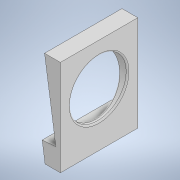
# Autodesk Inventor part: exhastForGasVent02
Saved by Autodesk Inventor 2021.1 (Build 251245000, 245)
## iProperties
Created: 2020-08-27
Part Number: exhastForGasVent02
Material: Generic
Document SubType Name: Modeling
Designer: robst
Density: 1 g/cm^3
Appearance: Default
Author: robst
Autodesk Inventor part; units mm, degrees
ref_plane "YZ Plane" through (0, 0, 0) normal (1, 0, 0) x (0, 1, 0)
ref_plane "XZ Plane" through (0, 0, 0) normal (0, 1, 0) x (-1, 0, 0)
ref_plane "XY Plane" through (0, 0, 0) normal (0, 0, 1) x (1, 0, 0)
sketch "Sketch6" plane through (0, 0, 0) normal (0, 0, 1) x (1, 0, 0)
  line L0 (0, 0) -> (0, 83.82)
  line L1 (0, 83.82) -> (-17.653, 83.82)
  line L2 (-17.653, 83.82) -> (-5.08, 0)
  line L3 (0, 0) -> (0, -22.86)
  line L4 (0, -22.86) -> (-17.091, -22.86)
  line L5 (-23.2881, 0) -> (-5.08, 0) construction
  line L6 (-5.08, 0) -> (-20.32, -1.3333)
  line L7 (-20.32, -1.3333) -> (-17.091, -22.86)
  dimension "d31" = 83.82
  dimension "d32" = 17.653
  dimension "d33" = 22.86
  dimension "d35" = 5
  dimension "d36" = 0
  dimension "d37" = 5.08
  dimension "d47" = 20.32
  constraints: 16 end point, 2 parallel, 2 perpendicular, 2 vertical
  measures "d31" distance of L0.start L0.end
  measures "d32" distance of L0.end L1.end
  measures "d33" distance of L0.start L3.end
  measures "d35" angle of L6 L5
  measures "d36" vertical distance of L2.end L0.start
  measures "d37" distance of L2.end L0.start
  measures "d47" distance from line of L6.end L3
extrude "Extrusion7" add sketch "Sketch6" along normal mid plane 86.36
sketch "Sketch7" plane through (0, -22.86, 43.18) normal (1, 0, 0) x (0, 0, -1)
  line L0 (86.36, 22.86) -> (0, 22.86) projected
  line L1 (0, 106.68) -> (86.36, 106.68) construction
  line L2 (43.18, 106.68) -> (43.18, 22.86) construction
  circle A0 centre (43.18, 59.69) radius 31.75
  dimension "d40" = 63.5
  dimension "d41" = 5.08
  constraints: 2 end point, 1 centre point, 1 midpoint, 1 perpendicular, 1 point on line
  measures "d40" diameter of A0
  measures "d41" distance edge to line of A0 L0
extrude "Extrusion8" cut sketch "Sketch7" against normal through all
sketch "Sketch11" plane through (-17.091, -22.86, -43.18) normal (-0.9889364, -0.1483405, 0) x (0, 0, 1)
  line L0 (43.18, 20.0718) -> (43.18, 0) construction
  line L1 (0, 0) -> (86.36, 0) construction
  line L2 (43.18, 10.0359) -> (86.36, 10.0359) construction
  spline S0 degree 2 poles (51.8782, 10.9729) (51.4467, 10.9729) (50.7321, 11.2363) (50.4752, 11.5031) knots 0 0 0 1 2 2 2
  spline S1 degree 2 poles (50.4752, 11.5031) (50.2183, 11.7731) (49.945, 12.5701) (49.945, 13.0872) knots 0 0 0 1 2 2 2
  spline S2 degree 2 poles (49.945, 13.0872) (49.945, 13.5779) (50.2216, 14.3551) (50.4785, 14.6318) knots 0 0 0 1 2 2 2
  spline S3 degree 2 poles (50.4785, 14.6318) (50.7255, 14.8985) (51.45, 15.1884) (51.8815, 15.1884) knots 0 0 0 1 2 2 2
  spline S4 degree 2 poles (51.8815, 15.1884) (52.0889, 15.1884) (52.4644, 15.1291) (52.6356, 15.0764) knots 0 0 0 1 2 2 2
  spline S5 degree 2 poles (52.6356, 15.0764) (52.774, 15.0369) (53.1099, 14.892) (53.212, 14.8393) knots 0 0 0 1 2 2 2
  line L3 (53.212, 14.8393) -> (53.212, 14.1872)
  line L4 (53.212, 14.1872) -> (53.1659, 14.1872)
  spline S6 degree 2 poles (53.1659, 14.1872) (53.0638, 14.2761) (52.8497, 14.4375) (52.6521, 14.5297) knots 0 0 0 1 2 2 2
  spline S7 degree 2 poles (52.6521, 14.5297) (52.4874, 14.612) (52.0626, 14.7207) (51.8189, 14.7207) knots 0 0 0 1 2 2 2
  spline S8 degree 2 poles (51.8189, 14.7207) (51.2327, 14.7207) (50.5081, 13.8381) (50.5081, 13.1037) knots 0 0 0 1 2 2 2
  spline S9 degree 2 poles (50.5081, 13.1037) (50.5081, 12.6953) (50.6991, 12.0827) (50.8803, 11.8719) knots 0 0 0 1 2 2 2
  spline S10 degree 2 poles (50.8803, 11.8719) (51.0548, 11.6612) (51.5488, 11.4405) (51.8584, 11.4405) knots 0 0 0 1 2 2 2
  spline S11 degree 2 poles (51.8584, 11.4405) (52.0856, 11.4405) (52.5401, 11.5064) (52.6949, 11.5722) knots 0 0 0 1 2 2 2
  line L5 (52.6949, 11.5722) -> (52.6949, 12.6228)
  line L6 (52.6949, 12.6228) -> (51.753, 12.6228)
  line L7 (51.753, 12.6228) -> (51.753, 13.0971)
  line L8 (51.753, 13.0971) -> (53.2284, 13.0971)
  line L9 (53.2284, 13.0971) -> (53.2284, 11.322)
  spline S12 degree 2 poles (53.2284, 11.322) (53.1263, 11.2758) (52.7772, 11.1342) (52.629, 11.0914) knots 0 0 0 1 2 2 2
  spline S13 degree 2 poles (52.629, 11.0914) (52.4282, 11.0321) (52.1054, 10.9729) (51.8782, 10.9729) knots 0 0 0 1 2 2 2
  spline S14 degree 2 poles (55.5667, 11.3746) (55.5041, 11.3285) (55.2934, 11.1639) (55.1946, 11.1145) knots 0 0 0 1 2 2 2
  spline S15 degree 2 poles (55.1946, 11.1145) (55.0595, 11.042) (54.806, 10.9663) (54.5754, 10.9663) knots 0 0 0 1 2 2 2
  spline S16 degree 2 poles (54.5754, 10.9663) (54.3877, 10.9663) (54.0485, 11.1079) (53.92, 11.2363) knots 0 0 0 1 2 2 2
  spline S17 degree 2 poles (53.92, 11.2363) (53.7982, 11.3615) (53.65, 11.7303) (53.65, 11.9345) knots 0 0 0 1 2 2 2
  spline S18 degree 2 poles (53.65, 11.9345) (53.65, 12.2507) (53.9167, 12.6986) (54.2066, 12.827) knots 0 0 0 1 2 2 2
  spline S19 degree 2 poles (54.2066, 12.827) (54.4634, 12.9456) (55.1616, 13.0345) (55.5667, 13.0576) knots 0 0 0 1 2 2 2
  line L10 (55.5667, 13.0576) -> (55.5667, 13.1564)
  spline S20 degree 2 poles (55.5667, 13.1564) (55.5667, 13.3342) (55.458, 13.5548) (55.3592, 13.6174) knots 0 0 0 1 2 2 2
  spline S21 degree 2 poles (55.3592, 13.6174) (55.2604, 13.68) (54.9772, 13.7195) (54.8257, 13.7195) knots 0 0 0 1 2 2 2
  spline S22 degree 2 poles (54.8257, 13.7195) (54.6479, 13.7195) (54.167, 13.6141) (53.9266, 13.512) knots 0 0 0 1 2 2 2
  line L11 (53.9266, 13.512) -> (53.897, 13.512)
  line L12 (53.897, 13.512) -> (53.897, 14.0357)
  spline S23 degree 2 poles (53.897, 14.0357) (54.0386, 14.0752) (54.5688, 14.174) (54.829, 14.174) knots 0 0 0 1 2 2 2
  spline S24 degree 2 poles (54.829, 14.174) (55.1452, 14.174) (55.5766, 14.0752) (55.7479, 13.9468) knots 0 0 0 1 2 2 2
  spline S25 degree 2 poles (55.7479, 13.9468) (55.9158, 13.8216) (56.0805, 13.4231) (56.0805, 13.1366) knots 0 0 0 1 2 2 2
  line L13 (56.0805, 13.1366) -> (56.0805, 11.0519)
  line L14 (56.0805, 11.0519) -> (55.5667, 11.0519)
  line L15 (55.5667, 11.0519) -> (55.5667, 11.3746)
  line L16 (55.5667, 11.8028) -> (55.5667, 12.6492)
  spline S26 degree 2 poles (55.5667, 12.6492) (55.3823, 12.6327) (54.8257, 12.5767) (54.6512, 12.524) knots 0 0 0 1 2 2 2
  spline S27 degree 2 poles (54.6512, 12.524) (54.447, 12.4615) (54.1802, 12.2013) (54.1802, 11.9707) knots 0 0 0 1 2 2 2
  spline S28 degree 2 poles (54.1802, 11.9707) (54.1802, 11.7073) (54.4766, 11.4405) (54.7598, 11.4405) knots 0 0 0 1 2 2 2
  spline S29 degree 2 poles (54.7598, 11.4405) (55.0003, 11.4405) (55.3955, 11.648) (55.5667, 11.8028) knots 0 0 0 1 2 2 2
  spline S30 degree 2 poles (57.6251, 10.9794) (57.3188, 10.9794) (56.7886, 11.1441) (56.614, 11.2363) knots 0 0 0 1 2 2 2
  line L17 (56.614, 11.2363) -> (56.614, 11.8127)
  line L18 (56.614, 11.8127) -> (56.6404, 11.8127)
  spline S31 degree 2 poles (56.6404, 11.8127) (56.7062, 11.76) (56.8841, 11.6348) (57.0323, 11.5657) knots 0 0 0 1 2 2 2
  spline S32 degree 2 poles (57.0323, 11.5657) (57.1607, 11.5031) (57.4769, 11.4109) (57.6448, 11.4109) knots 0 0 0 1 2 2 2
  spline S33 degree 2 poles (57.6448, 11.4109) (57.7667, 11.4109) (58.0466, 11.4669) (58.1125, 11.513) knots 0 0 0 1 2 2 2
  spline S34 degree 2 poles (58.1125, 11.513) (58.208, 11.5755) (58.2936, 11.7172) (58.2936, 11.8621) knots 0 0 0 1 2 2 2
  spline S35 degree 2 poles (58.2936, 11.8621) (58.2936, 12.0432) (58.096, 12.2309) (57.8424, 12.2935) knots 0 0 0 1 2 2 2
  spline S36 degree 2 poles (57.8424, 12.2935) (57.7436, 12.3165) (57.4275, 12.3824) (57.2924, 12.4186) knots 0 0 0 1 2 2 2
  spline S37 degree 2 poles (57.2924, 12.4186) (56.9433, 12.5207) (56.6272, 12.9423) (56.6272, 13.242) knots 0 0 0 1 2 2 2
  spline S38 degree 2 poles (56.6272, 13.242) (56.6272, 13.6569) (57.2496, 14.174) (57.7634, 14.174) knots 0 0 0 1 2 2 2
  spline S39 degree 2 poles (57.7634, 14.174) (58.017, 14.174) (58.5307, 14.0489) (58.7053, 13.9533) knots 0 0 0 1 2 2 2
  line L19 (58.7053, 13.9533) -> (58.7053, 13.4034)
  line L20 (58.7053, 13.4034) -> (58.6789, 13.4034)
  spline S40 degree 2 poles (58.6789, 13.4034) (58.4813, 13.5614) (58.0005, 13.7426) (57.7535, 13.7426) knots 0 0 0 1 2 2 2
  spline S41 degree 2 poles (57.7535, 13.7426) (57.4999, 13.7426) (57.1508, 13.5285) (57.1508, 13.3144) knots 0 0 0 1 2 2 2
  spline S42 degree 2 poles (57.1508, 13.3144) (57.1508, 13.1201) (57.3583, 12.9324) (57.5888, 12.8731) knots 0 0 0 1 2 2 2
  spline S43 degree 2 poles (57.5888, 12.8731) (57.7008, 12.8435) (57.984, 12.7842) (58.1388, 12.748) knots 0 0 0 1 2 2 2
  spline S44 degree 2 poles (58.1388, 12.748) (58.4748, 12.6623) (58.8173, 12.2704) (58.8173, 11.9312) knots 0 0 0 1 2 2 2
  spline S45 degree 2 poles (58.8173, 11.9312) (58.8173, 11.7336) (58.6625, 11.3845) (58.511, 11.2561) knots 0 0 0 1 2 2 2
  spline S46 degree 2 poles (58.511, 11.2561) (58.3496, 11.1211) (57.9379, 10.9794) (57.6251, 10.9794) knots 0 0 0 1 2 2 2
  line L21 (64.0273, 15.1159) -> (62.6277, 11.0519)
  line L22 (62.6277, 11.0519) -> (62.0447, 11.0519)
  line L23 (62.0447, 11.0519) -> (60.6451, 15.1159)
  line L24 (60.6451, 15.1159) -> (61.2247, 15.1159)
  line L25 (61.2247, 15.1159) -> (62.351, 11.7402)
  line L26 (62.351, 11.7402) -> (63.4774, 15.1159)
  line L27 (63.4774, 15.1159) -> (64.0273, 15.1159)
  spline S47 degree 2 poles (65.7465, 10.9827) (65.0154, 10.9827) (64.2118, 11.8028) (64.2118, 12.5603) knots 0 0 0 1 2 2 2
  spline S48 degree 2 poles (64.2118, 12.5603) (64.2118, 13.3046) (64.9923, 14.1872) (65.6213, 14.1872) knots 0 0 0 1 2 2 2
  spline S49 degree 2 poles (65.6213, 14.1872) (65.9046, 14.1872) (66.3426, 14.0225) (66.504, 13.848) knots 0 0 0 1 2 2 2
  spline S50 degree 2 poles (66.504, 13.848) (66.6686, 13.6734) (66.8432, 13.1695) (66.8432, 12.804) knots 0 0 0 1 2 2 2
  line L28 (66.8432, 12.804) -> (66.8432, 12.524)
  line L29 (66.8432, 12.524) -> (64.7321, 12.524)
  spline S51 degree 2 poles (64.7321, 12.524) (64.7321, 11.9938) (65.2656, 11.4306) (65.7399, 11.4306) knots 0 0 0 1 2 2 2
  spline S52 degree 2 poles (65.7399, 11.4306) (65.9079, 11.4306) (66.2339, 11.5064) (66.3656, 11.5657) knots 0 0 0 1 2 2 2
  spline S53 degree 2 poles (66.3656, 11.5657) (66.504, 11.6315) (66.695, 11.7468) (66.7575, 11.7995) knots 0 0 0 1 2 2 2
  line L30 (66.7575, 11.7995) -> (66.7872, 11.7995)
  line L31 (66.7872, 11.7995) -> (66.7872, 11.2396)
  spline S54 degree 2 poles (66.7872, 11.2396) (66.6983, 11.2034) (66.4282, 11.098) (66.3228, 11.0684) knots 0 0 0 1 2 2 2
  spline S55 degree 2 poles (66.3228, 11.0684) (66.1746, 11.0256) (65.9309, 10.9827) (65.7465, 10.9827) knots 0 0 0 1 2 2 2
  spline S56 degree 2 poles (66.3426, 12.9159) (66.336, 13.1234) (66.2504, 13.4264) (66.168, 13.5285) knots 0 0 0 1 2 2 2
  spline S57 degree 2 poles (66.168, 13.5285) (66.0791, 13.6438) (65.7992, 13.7656) (65.5917, 13.7656) knots 0 0 0 1 2 2 2
  spline S58 degree 2 poles (65.5917, 13.7656) (65.3875, 13.7656) (65.101, 13.6438) (64.9824, 13.5252) knots 0 0 0 1 2 2 2
  spline S59 degree 2 poles (64.9824, 13.5252) (64.8672, 13.4034) (64.7486, 13.1102) (64.7321, 12.9159) knots 0 0 0 1 2 2 2
  line L32 (64.7321, 12.9159) -> (66.3426, 12.9159)
  line L33 (69.7578, 11.0519) -> (69.244, 11.0519)
  line L34 (69.244, 11.0519) -> (69.244, 12.7908)
  spline S60 degree 2 poles (69.244, 12.7908) (69.244, 13.0016) (69.2045, 13.3638) (69.1452, 13.4725) knots 0 0 0 1 2 2 2
  spline S61 degree 2 poles (69.1452, 13.4725) (69.0826, 13.5878) (68.8587, 13.6998) (68.6677, 13.6998) knots 0 0 0 1 2 2 2
  spline S62 degree 2 poles (68.6677, 13.6998) (68.4767, 13.6998) (68.0716, 13.4956) (67.8773, 13.3309) knots 0 0 0 1 2 2 2
  line L35 (67.8773, 13.3309) -> (67.8773, 11.0519)
  line L36 (67.8773, 11.0519) -> (67.3635, 11.0519)
  line L37 (67.3635, 11.0519) -> (67.3635, 14.1015)
  line L38 (67.3635, 14.1015) -> (67.8773, 14.1015)
  line L39 (67.8773, 14.1015) -> (67.8773, 13.7623)
  spline S63 degree 2 poles (67.8773, 13.7623) (68.1078, 13.9698) (68.5524, 14.1872) (68.8027, 14.1872) knots 0 0 0 1 2 2 2
  spline S64 degree 2 poles (68.8027, 14.1872) (69.2506, 14.1872) (69.7578, 13.5944) (69.7578, 13.0312) knots 0 0 0 1 2 2 2
  line L40 (69.7578, 13.0312) -> (69.7578, 11.0519)
  spline S65 degree 2 poles (71.4012, 10.9926) (70.9829, 10.9926) (70.512, 11.4702) (70.512, 11.9872) knots 0 0 0 1 2 2 2
  line L41 (70.512, 11.9872) -> (70.512, 13.6767)
  line L42 (70.512, 13.6767) -> (70.1662, 13.6767)
  line L43 (70.1662, 13.6767) -> (70.1662, 14.1015)
  line L44 (70.1662, 14.1015) -> (70.512, 14.1015)
  line L45 (70.512, 14.1015) -> (70.512, 14.9776)
  line L46 (70.512, 14.9776) -> (71.0257, 14.9776)
  line L47 (71.0257, 14.9776) -> (71.0257, 14.1015)
  line L48 (71.0257, 14.1015) -> (71.9709, 14.1015)
  line L49 (71.9709, 14.1015) -> (71.9709, 13.6767)
  line L50 (71.9709, 13.6767) -> (71.0257, 13.6767)
  line L51 (71.0257, 13.6767) -> (71.0257, 12.2243)
  spline S66 degree 2 poles (71.0257, 12.2243) (71.0257, 11.9938) (71.0422, 11.7402) (71.0982, 11.6315) knots 0 0 0 1 2 2 2
  spline S67 degree 2 poles (71.0982, 11.6315) (71.1443, 11.536) (71.3518, 11.4405) (71.5296, 11.4405) knots 0 0 0 1 2 2 2
  spline S68 degree 2 poles (71.5296, 11.4405) (71.6548, 11.4405) (71.8886, 11.5163) (71.9413, 11.5393) knots 0 0 0 1 2 2 2
  line L52 (71.9413, 11.5393) -> (71.9709, 11.5393)
  line L53 (71.9709, 11.5393) -> (71.9709, 11.0782)
  spline S69 degree 2 poles (71.9709, 11.0782) (71.826, 11.0387) (71.5296, 10.9926) (71.4012, 10.9926) knots 0 0 0 1 2 2 2
  spline S70 degree 2 poles (76.5487, 13.0839) (76.5487, 11.9905) (75.9131, 10.9663) (75.2511, 10.9663) knots 0 0 0 1 2 2 2
  spline S71 degree 2 poles (75.2511, 10.9663) (74.5793, 10.9663) (73.9502, 12.0103) (73.9502, 13.0806) knots 0 0 0 1 2 2 2
  spline S72 degree 2 poles (73.9502, 13.0806) (73.9502, 14.1806) (74.5858, 15.1982) (75.2511, 15.1982) knots 0 0 0 1 2 2 2
  spline S73 degree 2 poles (75.2511, 15.1982) (75.9197, 15.1982) (76.5487, 14.1444) (76.5487, 13.0839) knots 0 0 0 1 2 2 2
  spline S74 degree 2 poles (75.8505, 11.8456) (75.9295, 12.0465) (75.9954, 12.6656) (75.9954, 13.0839) knots 0 0 0 1 2 2 2
  spline S75 degree 2 poles (75.9954, 13.0839) (75.9954, 13.5022) (75.9295, 14.118) (75.8472, 14.3255) knots 0 0 0 1 2 2 2
  spline S76 degree 2 poles (75.8472, 14.3255) (75.7649, 14.533) (75.4783, 14.747) (75.2511, 14.747) knots 0 0 0 1 2 2 2
  spline S77 degree 2 poles (75.2511, 14.747) (75.0239, 14.747) (74.7308, 14.533) (74.6451, 14.3189) knots 0 0 0 1 2 2 2
  spline S78 degree 2 poles (74.6451, 14.3189) (74.5628, 14.1114) (74.5035, 13.4791) (74.5035, 13.0806) knots 0 0 0 1 2 2 2
  spline S79 degree 2 poles (74.5035, 13.0806) (74.5035, 12.6525) (74.5562, 12.0794) (74.6418, 11.8555) knots 0 0 0 1 2 2 2
  spline S80 degree 2 poles (74.6418, 11.8555) (74.7209, 11.6447) (75.014, 11.4175) (75.2511, 11.4175) knots 0 0 0 1 2 2 2
  spline S81 degree 2 poles (75.2511, 11.4175) (75.475, 11.4175) (75.7682, 11.6315) (75.8505, 11.8456) knots 0 0 0 1 2 2 2
  line L54 (79.5753, 11.0519) -> (77.069, 11.0519)
  line L55 (77.069, 11.0519) -> (77.069, 11.6282)
  spline S82 degree 2 poles (77.069, 11.6282) (77.3391, 11.8818) (77.8199, 12.3528) (78.0505, 12.6064) knots 0 0 0 1 2 2 2
  spline S83 degree 2 poles (78.0505, 12.6064) (78.5148, 13.1168) (78.854, 13.7294) (78.854, 14.0554) knots 0 0 0 1 2 2 2
  spline S84 degree 2 poles (78.854, 14.0554) (78.854, 14.2267) (78.7486, 14.4836) (78.6531, 14.5659) knots 0 0 0 1 2 2 2
  spline S85 degree 2 poles (78.6531, 14.5659) (78.5576, 14.6482) (78.3073, 14.7306) (78.1558, 14.7306) knots 0 0 0 1 2 2 2
  spline S86 degree 2 poles (78.1558, 14.7306) (78.0109, 14.7306) (77.7145, 14.6581) (77.5795, 14.6021) knots 0 0 0 1 2 2 2
  spline S87 degree 2 poles (77.5795, 14.6021) (77.4642, 14.556) (77.2502, 14.4243) (77.1843, 14.3782) knots 0 0 0 1 2 2 2
  line L56 (77.1843, 14.3782) -> (77.1547, 14.3782)
  line L57 (77.1547, 14.3782) -> (77.1547, 14.9578)
  spline S88 degree 2 poles (77.1547, 14.9578) (77.3226, 15.0402) (77.9253, 15.2015) (78.1954, 15.2015) knots 0 0 0 1 2 2 2
  spline S89 degree 2 poles (78.1954, 15.2015) (78.7651, 15.2015) (79.4073, 14.5988) (79.4073, 14.0851) knots 0 0 0 1 2 2 2
  spline S90 degree 2 poles (79.4073, 14.0851) (79.4073, 13.8447) (79.2953, 13.4429) (79.1965, 13.2716) knots 0 0 0 1 2 2 2
  spline S91 degree 2 poles (79.1965, 13.2716) (79.0977, 13.0938) (78.8112, 12.7447) (78.6531, 12.5767) knots 0 0 0 1 2 2 2
  spline S92 degree 2 poles (78.6531, 12.5767) (78.3963, 12.2968) (77.7672, 11.6974) (77.5795, 11.5228) knots 0 0 0 1 2 2 2
  line L58 (77.5795, 11.5228) -> (79.5753, 11.5228)
  line L59 (79.5753, 11.5228) -> (79.5753, 11.0519)
  spline S93 degree 2 poles (55.4646, 7.1796) (55.4646, 6.9162) (55.2769, 6.4419) (55.1089, 6.2773) knots 0 0 0 1 2 2 2
  spline S94 degree 2 poles (55.1089, 6.2773) (54.8982, 6.0698) (54.3284, 5.8557) (53.8937, 5.8557) knots 0 0 0 1 2 2 2
  line L60 (53.8937, 5.8557) -> (53.4359, 5.8557)
  line L61 (53.4359, 5.8557) -> (53.4359, 4.3408)
  line L62 (53.4359, 4.3408) -> (52.8958, 4.3408)
  line L63 (52.8958, 4.3408) -> (52.8958, 8.4048)
  line L64 (52.8958, 8.4048) -> (53.9167, 8.4048)
  spline S95 degree 2 poles (53.9167, 8.4048) (54.279, 8.4048) (54.7862, 8.2862) (54.9805, 8.1512) knots 0 0 0 1 2 2 2
  spline S96 degree 2 poles (54.9805, 8.1512) (55.2077, 7.9964) (55.4646, 7.5189) (55.4646, 7.1796) knots 0 0 0 1 2 2 2
  spline S97 degree 2 poles (54.9015, 7.1632) (54.9015, 7.374) (54.7566, 7.6835) (54.6084, 7.7823) knots 0 0 0 1 2 2 2
  spline S98 degree 2 poles (54.6084, 7.7823) (54.4799, 7.868) (54.1374, 7.9371) (53.8838, 7.9371) knots 0 0 0 1 2 2 2
  line L65 (53.8838, 7.9371) -> (53.4359, 7.9371)
  line L66 (53.4359, 7.9371) -> (53.4359, 6.3168)
  line L67 (53.4359, 6.3168) -> (53.8048, 6.3168)
  spline S99 degree 2 poles (53.8048, 6.3168) (54.1341, 6.3168) (54.5392, 6.4222) (54.6709, 6.5605) knots 0 0 0 1 2 2 2
  spline S100 degree 2 poles (54.6709, 6.5605) (54.7928, 6.6824) (54.9015, 6.9689) (54.9015, 7.1632) knots 0 0 0 1 2 2 2
  line L68 (57.5559, 6.8404) -> (57.5296, 6.8404)
  spline S101 degree 2 poles (57.5296, 6.8404) (57.4703, 6.8569) (57.3418, 6.8635) (57.2529, 6.8635) knots 0 0 0 1 2 2 2
  spline S102 degree 2 poles (57.2529, 6.8635) (57.0454, 6.8635) (56.6371, 6.6824) (56.4526, 6.5045) knots 0 0 0 1 2 2 2
  line L69 (56.4526, 6.5045) -> (56.4526, 4.3408)
  line L70 (56.4526, 4.3408) -> (55.9389, 4.3408)
  line L71 (55.9389, 4.3408) -> (55.9389, 7.3904)
  line L72 (55.9389, 7.3904) -> (56.4526, 7.3904)
  line L73 (56.4526, 7.3904) -> (56.4526, 6.9359)
  spline S103 degree 2 poles (56.4526, 6.9359) (56.7326, 7.1862) (57.1508, 7.3904) (57.3484, 7.3904) knots 0 0 0 1 2 2 2
  spline S104 degree 2 poles (57.3484, 7.3904) (57.4275, 7.3904) (57.5065, 7.3838) (57.5559, 7.374) knots 0 0 0 1 2 2 2
  line L74 (57.5559, 7.374) -> (57.5559, 6.8404)
  line L75 (58.478, 4.3408) -> (57.9643, 4.3408)
  line L76 (57.9643, 4.3408) -> (57.9643, 7.3904)
  line L77 (57.9643, 7.3904) -> (58.478, 7.3904)
  line L78 (58.478, 7.3904) -> (58.478, 4.3408)
  line L79 (58.5143, 7.8976) -> (57.9313, 7.8976)
  line L80 (57.9313, 7.8976) -> (57.9313, 8.4311)
  line L81 (57.9313, 8.4311) -> (58.5143, 8.4311)
  line L82 (58.5143, 8.4311) -> (58.5143, 7.8976)
  line L83 (61.6265, 4.3408) -> (61.1127, 4.3408)
  line L84 (61.1127, 4.3408) -> (61.1127, 6.0797)
  spline S105 degree 2 poles (61.1127, 6.0797) (61.1127, 6.2904) (61.0732, 6.6527) (61.0139, 6.7614) knots 0 0 0 1 2 2 2
  spline S106 degree 2 poles (61.0139, 6.7614) (60.9514, 6.8767) (60.7274, 6.9886) (60.5364, 6.9886) knots 0 0 0 1 2 2 2
  spline S107 degree 2 poles (60.5364, 6.9886) (60.3454, 6.9886) (59.9403, 6.7844) (59.746, 6.6198) knots 0 0 0 1 2 2 2
  line L85 (59.746, 6.6198) -> (59.746, 4.3408)
  line L86 (59.746, 4.3408) -> (59.2322, 4.3408)
  line L87 (59.2322, 4.3408) -> (59.2322, 7.3904)
  line L88 (59.2322, 7.3904) -> (59.746, 7.3904)
  line L89 (59.746, 7.3904) -> (59.746, 7.0512)
  spline S108 degree 2 poles (59.746, 7.0512) (59.9765, 7.2587) (60.4211, 7.476) (60.6714, 7.476) knots 0 0 0 1 2 2 2
  spline S109 degree 2 poles (60.6714, 7.476) (61.1193, 7.476) (61.6265, 6.8832) (61.6265, 6.3201) knots 0 0 0 1 2 2 2
  line L90 (61.6265, 6.3201) -> (61.6265, 4.3408)
  spline S110 degree 2 poles (63.2699, 4.2815) (62.8516, 4.2815) (62.3807, 4.759) (62.3807, 5.2761) knots 0 0 0 1 2 2 2
  line L91 (62.3807, 5.2761) -> (62.3807, 6.9656)
  line L92 (62.3807, 6.9656) -> (62.0349, 6.9656)
  line L93 (62.0349, 6.9656) -> (62.0349, 7.3904)
  line L94 (62.0349, 7.3904) -> (62.3807, 7.3904)
  line L95 (62.3807, 7.3904) -> (62.3807, 8.2665)
  line L96 (62.3807, 8.2665) -> (62.8944, 8.2665)
  line L97 (62.8944, 8.2665) -> (62.8944, 7.3904)
  line L98 (62.8944, 7.3904) -> (63.8396, 7.3904)
  line L99 (63.8396, 7.3904) -> (63.8396, 6.9656)
  line L100 (63.8396, 6.9656) -> (62.8944, 6.9656)
  line L101 (62.8944, 6.9656) -> (62.8944, 5.5132)
  spline S111 degree 2 poles (62.8944, 5.5132) (62.8944, 5.2827) (62.9109, 5.0291) (62.9669, 4.9204) knots 0 0 0 1 2 2 2
  spline S112 degree 2 poles (62.9669, 4.9204) (63.013, 4.8249) (63.2205, 4.7294) (63.3983, 4.7294) knots 0 0 0 1 2 2 2
  spline S113 degree 2 poles (63.3983, 4.7294) (63.5235, 4.7294) (63.7573, 4.8051) (63.81, 4.8282) knots 0 0 0 1 2 2 2
  line L102 (63.81, 4.8282) -> (63.8396, 4.8282)
  line L103 (63.8396, 4.8282) -> (63.8396, 4.3671)
  spline S114 degree 2 poles (63.8396, 4.3671) (63.6947, 4.3276) (63.3983, 4.2815) (63.2699, 4.2815) knots 0 0 0 1 2 2 2
  line L104 (68.9509, 8.4048) -> (67.5512, 4.3408)
  line L105 (67.5512, 4.3408) -> (66.9683, 4.3408)
  line L106 (66.9683, 4.3408) -> (65.5686, 8.4048)
  line L107 (65.5686, 8.4048) -> (66.1483, 8.4048)
  line L108 (66.1483, 8.4048) -> (67.2746, 5.0291)
  line L109 (67.2746, 5.0291) -> (68.4009, 8.4048)
  line L110 (68.4009, 8.4048) -> (68.9509, 8.4048)
  line L111 (70.759, 5.8722) -> (69.221, 5.8722)
  line L112 (69.221, 5.8722) -> (69.221, 6.3662)
  line L113 (69.221, 6.3662) -> (70.759, 6.3662)
  line L114 (70.759, 6.3662) -> (70.759, 5.8722)
  spline S115 degree 2 poles (73.8284, 6.3728) (73.8284, 5.2794) (73.1928, 4.2551) (72.5308, 4.2551) knots 0 0 0 1 2 2 2
  spline S116 degree 2 poles (72.5308, 4.2551) (71.8589, 4.2551) (71.2299, 5.2991) (71.2299, 6.3695) knots 0 0 0 1 2 2 2
  spline S117 degree 2 poles (71.2299, 6.3695) (71.2299, 7.4695) (71.8655, 8.4871) (72.5308, 8.4871) knots 0 0 0 1 2 2 2
  spline S118 degree 2 poles (72.5308, 8.4871) (73.1993, 8.4871) (73.8284, 7.4332) (73.8284, 6.3728) knots 0 0 0 1 2 2 2
  spline S119 degree 2 poles (73.1302, 5.1345) (73.2092, 5.3354) (73.2751, 5.9545) (73.2751, 6.3728) knots 0 0 0 1 2 2 2
  spline S120 degree 2 poles (73.2751, 6.3728) (73.2751, 6.791) (73.2092, 7.4069) (73.1269, 7.6144) knots 0 0 0 1 2 2 2
  spline S121 degree 2 poles (73.1269, 7.6144) (73.0446, 7.8219) (72.758, 8.0359) (72.5308, 8.0359) knots 0 0 0 1 2 2 2
  spline S122 degree 2 poles (72.5308, 8.0359) (72.3035, 8.0359) (72.0104, 7.8219) (71.9248, 7.6078) knots 0 0 0 1 2 2 2
  spline S123 degree 2 poles (71.9248, 7.6078) (71.8425, 7.4003) (71.7832, 6.768) (71.7832, 6.3695) knots 0 0 0 1 2 2 2
  spline S124 degree 2 poles (71.7832, 6.3695) (71.7832, 5.9413) (71.8359, 5.3683) (71.9215, 5.1444) knots 0 0 0 1 2 2 2
  spline S125 degree 2 poles (71.9215, 5.1444) (72.0006, 4.9336) (72.2937, 4.7063) (72.5308, 4.7063) knots 0 0 0 1 2 2 2
  spline S126 degree 2 poles (72.5308, 4.7063) (72.7547, 4.7063) (73.0478, 4.9204) (73.1302, 5.1345) knots 0 0 0 1 2 2 2
  line L115 (76.855, 4.3408) -> (74.3487, 4.3408)
  line L116 (74.3487, 4.3408) -> (74.3487, 4.9171)
  spline S127 degree 2 poles (74.3487, 4.9171) (74.6188, 5.1707) (75.0996, 5.6417) (75.3301, 5.8952) knots 0 0 0 1 2 2 2
  spline S128 degree 2 poles (75.3301, 5.8952) (75.7945, 6.4057) (76.1337, 7.0183) (76.1337, 7.3443) knots 0 0 0 1 2 2 2
  spline S129 degree 2 poles (76.1337, 7.3443) (76.1337, 7.5156) (76.0283, 7.7725) (75.9328, 7.8548) knots 0 0 0 1 2 2 2
  spline S130 degree 2 poles (75.9328, 7.8548) (75.8373, 7.9371) (75.587, 8.0195) (75.4355, 8.0195) knots 0 0 0 1 2 2 2
  spline S131 degree 2 poles (75.4355, 8.0195) (75.2906, 8.0195) (74.9942, 7.947) (74.8592, 7.891) knots 0 0 0 1 2 2 2
  spline S132 degree 2 poles (74.8592, 7.891) (74.7439, 7.8449) (74.5299, 7.7132) (74.464, 7.6671) knots 0 0 0 1 2 2 2
  line L117 (74.464, 7.6671) -> (74.4344, 7.6671)
  line L118 (74.4344, 7.6671) -> (74.4344, 8.2467)
  spline S133 degree 2 poles (74.4344, 8.2467) (74.6023, 8.329) (75.205, 8.4904) (75.4751, 8.4904) knots 0 0 0 1 2 2 2
  spline S134 degree 2 poles (75.4751, 8.4904) (76.0448, 8.4904) (76.687, 7.8877) (76.687, 7.374) knots 0 0 0 1 2 2 2
  spline S135 degree 2 poles (76.687, 7.374) (76.687, 7.1335) (76.575, 6.7318) (76.4762, 6.5605) knots 0 0 0 1 2 2 2
  spline S136 degree 2 poles (76.4762, 6.5605) (76.3774, 6.3827) (76.0909, 6.0336) (75.9328, 5.8656) knots 0 0 0 1 2 2 2
  spline S137 degree 2 poles (75.9328, 5.8656) (75.6759, 5.5857) (75.0469, 4.9863) (74.8592, 4.8117) knots 0 0 0 1 2 2 2
  line L119 (74.8592, 4.8117) -> (76.855, 4.8117)
  line L120 (76.855, 4.8117) -> (76.855, 4.3408)
  constraints: 4 end point, 2 horizontal, 2 midpoint
extrude "Extrusion11" cut sketch "Sketch11" against normal blind 1.27
fillet "Fillet1" radius 1.5875 2 edges at (0, 36.83, 31.75) (-10.6045, 36.83, 31.75)
sketch "Sketch12" plane through (-17.091, -22.86, -43.18) normal (-0.9889364, -0.1483405, 0) x (0, 0, 1)
  line L0 (43.18, 20.0718) -> (43.18, 0) construction
  line L1 (0, 0) -> (86.36, 0) construction
  line L2 (43.18, 10.0359) -> (0, 10.0359) construction
  line L3 (0, 0) -> (0, 21.7675) construction
  spline S0 degree 2 poles (8.6982, 10.9729) (8.2667, 10.9729) (7.5521, 11.2363) (7.2952, 11.5031) knots 0 0 0 1 2 2 2
  spline S1 degree 2 poles (7.2952, 11.5031) (7.0383, 11.7731) (6.765, 12.5701) (6.765, 13.0872) knots 0 0 0 1 2 2 2
  spline S2 degree 2 poles (6.765, 13.0872) (6.765, 13.5779) (7.0416, 14.3551) (7.2985, 14.6318) knots 0 0 0 1 2 2 2
  spline S3 degree 2 poles (7.2985, 14.6318) (7.5455, 14.8985) (8.27, 15.1884) (8.7015, 15.1884) knots 0 0 0 1 2 2 2
  spline S4 degree 2 poles (8.7015, 15.1884) (8.9089, 15.1884) (9.2844, 15.1291) (9.4556, 15.0764) knots 0 0 0 1 2 2 2
  spline S5 degree 2 poles (9.4556, 15.0764) (9.594, 15.0369) (9.9299, 14.892) (10.032, 14.8393) knots 0 0 0 1 2 2 2
  line L4 (10.032, 14.8393) -> (10.032, 14.1872)
  line L5 (10.032, 14.1872) -> (9.9859, 14.1872)
  spline S6 degree 2 poles (9.9859, 14.1872) (9.8838, 14.2761) (9.6697, 14.4375) (9.4721, 14.5297) knots 0 0 0 1 2 2 2
  spline S7 degree 2 poles (9.4721, 14.5297) (9.3074, 14.612) (8.8826, 14.7207) (8.6389, 14.7207) knots 0 0 0 1 2 2 2
  spline S8 degree 2 poles (8.6389, 14.7207) (8.0527, 14.7207) (7.3281, 13.8381) (7.3281, 13.1037) knots 0 0 0 1 2 2 2
  spline S9 degree 2 poles (7.3281, 13.1037) (7.3281, 12.6953) (7.5191, 12.0827) (7.7003, 11.8719) knots 0 0 0 1 2 2 2
  spline S10 degree 2 poles (7.7003, 11.8719) (7.8748, 11.6612) (8.3688, 11.4405) (8.6784, 11.4405) knots 0 0 0 1 2 2 2
  spline S11 degree 2 poles (8.6784, 11.4405) (8.9056, 11.4405) (9.3601, 11.5064) (9.5149, 11.5722) knots 0 0 0 1 2 2 2
  line L6 (9.5149, 11.5722) -> (9.5149, 12.6228)
  line L7 (9.5149, 12.6228) -> (8.573, 12.6228)
  line L8 (8.573, 12.6228) -> (8.573, 13.0971)
  line L9 (8.573, 13.0971) -> (10.0484, 13.0971)
  line L10 (10.0484, 13.0971) -> (10.0484, 11.322)
  spline S12 degree 2 poles (10.0484, 11.322) (9.9463, 11.2758) (9.5972, 11.1342) (9.449, 11.0914) knots 0 0 0 1 2 2 2
  spline S13 degree 2 poles (9.449, 11.0914) (9.2482, 11.0321) (8.9254, 10.9729) (8.6982, 10.9729) knots 0 0 0 1 2 2 2
  spline S14 degree 2 poles (12.3867, 11.3746) (12.3241, 11.3285) (12.1134, 11.1639) (12.0146, 11.1145) knots 0 0 0 1 2 2 2
  spline S15 degree 2 poles (12.0146, 11.1145) (11.8795, 11.042) (11.626, 10.9663) (11.3954, 10.9663) knots 0 0 0 1 2 2 2
  spline S16 degree 2 poles (11.3954, 10.9663) (11.2077, 10.9663) (10.8685, 11.1079) (10.74, 11.2363) knots 0 0 0 1 2 2 2
  spline S17 degree 2 poles (10.74, 11.2363) (10.6182, 11.3615) (10.47, 11.7303) (10.47, 11.9345) knots 0 0 0 1 2 2 2
  spline S18 degree 2 poles (10.47, 11.9345) (10.47, 12.2507) (10.7367, 12.6986) (11.0266, 12.827) knots 0 0 0 1 2 2 2
  spline S19 degree 2 poles (11.0266, 12.827) (11.2834, 12.9456) (11.9816, 13.0345) (12.3867, 13.0576) knots 0 0 0 1 2 2 2
  line L11 (12.3867, 13.0576) -> (12.3867, 13.1564)
  spline S20 degree 2 poles (12.3867, 13.1564) (12.3867, 13.3342) (12.278, 13.5548) (12.1792, 13.6174) knots 0 0 0 1 2 2 2
  spline S21 degree 2 poles (12.1792, 13.6174) (12.0804, 13.68) (11.7972, 13.7195) (11.6457, 13.7195) knots 0 0 0 1 2 2 2
  spline S22 degree 2 poles (11.6457, 13.7195) (11.4679, 13.7195) (10.987, 13.6141) (10.7466, 13.512) knots 0 0 0 1 2 2 2
  line L12 (10.7466, 13.512) -> (10.717, 13.512)
  line L13 (10.717, 13.512) -> (10.717, 14.0357)
  spline S23 degree 2 poles (10.717, 14.0357) (10.8586, 14.0752) (11.3888, 14.174) (11.649, 14.174) knots 0 0 0 1 2 2 2
  spline S24 degree 2 poles (11.649, 14.174) (11.9652, 14.174) (12.3966, 14.0752) (12.5679, 13.9468) knots 0 0 0 1 2 2 2
  spline S25 degree 2 poles (12.5679, 13.9468) (12.7358, 13.8216) (12.9005, 13.4231) (12.9005, 13.1366) knots 0 0 0 1 2 2 2
  line L14 (12.9005, 13.1366) -> (12.9005, 11.0519)
  line L15 (12.9005, 11.0519) -> (12.3867, 11.0519)
  line L16 (12.3867, 11.0519) -> (12.3867, 11.3746)
  line L17 (12.3867, 11.8028) -> (12.3867, 12.6492)
  spline S26 degree 2 poles (12.3867, 12.6492) (12.2023, 12.6327) (11.6457, 12.5767) (11.4712, 12.524) knots 0 0 0 1 2 2 2
  spline S27 degree 2 poles (11.4712, 12.524) (11.267, 12.4615) (11.0002, 12.2013) (11.0002, 11.9707) knots 0 0 0 1 2 2 2
  spline S28 degree 2 poles (11.0002, 11.9707) (11.0002, 11.7073) (11.2966, 11.4405) (11.5798, 11.4405) knots 0 0 0 1 2 2 2
  spline S29 degree 2 poles (11.5798, 11.4405) (11.8203, 11.4405) (12.2155, 11.648) (12.3867, 11.8028) knots 0 0 0 1 2 2 2
  spline S30 degree 2 poles (14.4451, 10.9794) (14.1388, 10.9794) (13.6086, 11.1441) (13.434, 11.2363) knots 0 0 0 1 2 2 2
  line L18 (13.434, 11.2363) -> (13.434, 11.8127)
  line L19 (13.434, 11.8127) -> (13.4604, 11.8127)
  spline S31 degree 2 poles (13.4604, 11.8127) (13.5262, 11.76) (13.7041, 11.6348) (13.8523, 11.5657) knots 0 0 0 1 2 2 2
  spline S32 degree 2 poles (13.8523, 11.5657) (13.9807, 11.5031) (14.2969, 11.4109) (14.4648, 11.4109) knots 0 0 0 1 2 2 2
  spline S33 degree 2 poles (14.4648, 11.4109) (14.5867, 11.4109) (14.8666, 11.4669) (14.9325, 11.513) knots 0 0 0 1 2 2 2
  spline S34 degree 2 poles (14.9325, 11.513) (15.028, 11.5755) (15.1136, 11.7172) (15.1136, 11.8621) knots 0 0 0 1 2 2 2
  spline S35 degree 2 poles (15.1136, 11.8621) (15.1136, 12.0432) (14.916, 12.2309) (14.6624, 12.2935) knots 0 0 0 1 2 2 2
  spline S36 degree 2 poles (14.6624, 12.2935) (14.5636, 12.3165) (14.2475, 12.3824) (14.1124, 12.4186) knots 0 0 0 1 2 2 2
  spline S37 degree 2 poles (14.1124, 12.4186) (13.7633, 12.5207) (13.4472, 12.9423) (13.4472, 13.242) knots 0 0 0 1 2 2 2
  spline S38 degree 2 poles (13.4472, 13.242) (13.4472, 13.6569) (14.0696, 14.174) (14.5834, 14.174) knots 0 0 0 1 2 2 2
  spline S39 degree 2 poles (14.5834, 14.174) (14.837, 14.174) (15.3507, 14.0489) (15.5253, 13.9533) knots 0 0 0 1 2 2 2
  line L20 (15.5253, 13.9533) -> (15.5253, 13.4034)
  line L21 (15.5253, 13.4034) -> (15.4989, 13.4034)
  spline S40 degree 2 poles (15.4989, 13.4034) (15.3013, 13.5614) (14.8205, 13.7426) (14.5735, 13.7426) knots 0 0 0 1 2 2 2
  spline S41 degree 2 poles (14.5735, 13.7426) (14.3199, 13.7426) (13.9708, 13.5285) (13.9708, 13.3144) knots 0 0 0 1 2 2 2
  spline S42 degree 2 poles (13.9708, 13.3144) (13.9708, 13.1201) (14.1783, 12.9324) (14.4088, 12.8731) knots 0 0 0 1 2 2 2
  spline S43 degree 2 poles (14.4088, 12.8731) (14.5208, 12.8435) (14.804, 12.7842) (14.9588, 12.748) knots 0 0 0 1 2 2 2
  spline S44 degree 2 poles (14.9588, 12.748) (15.2948, 12.6623) (15.6373, 12.2704) (15.6373, 11.9312) knots 0 0 0 1 2 2 2
  spline S45 degree 2 poles (15.6373, 11.9312) (15.6373, 11.7336) (15.4825, 11.3845) (15.331, 11.2561) knots 0 0 0 1 2 2 2
  spline S46 degree 2 poles (15.331, 11.2561) (15.1696, 11.1211) (14.7579, 10.9794) (14.4451, 10.9794) knots 0 0 0 1 2 2 2
  line L22 (20.8473, 15.1159) -> (19.4477, 11.0519)
  line L23 (19.4477, 11.0519) -> (18.8647, 11.0519)
  line L24 (18.8647, 11.0519) -> (17.4651, 15.1159)
  line L25 (17.4651, 15.1159) -> (18.0447, 15.1159)
  line L26 (18.0447, 15.1159) -> (19.171, 11.7402)
  line L27 (19.171, 11.7402) -> (20.2974, 15.1159)
  line L28 (20.2974, 15.1159) -> (20.8473, 15.1159)
  spline S47 degree 2 poles (22.5665, 10.9827) (21.8354, 10.9827) (21.0318, 11.8028) (21.0318, 12.5603) knots 0 0 0 1 2 2 2
  spline S48 degree 2 poles (21.0318, 12.5603) (21.0318, 13.3046) (21.8123, 14.1872) (22.4413, 14.1872) knots 0 0 0 1 2 2 2
  spline S49 degree 2 poles (22.4413, 14.1872) (22.7246, 14.1872) (23.1626, 14.0225) (23.324, 13.848) knots 0 0 0 1 2 2 2
  spline S50 degree 2 poles (23.324, 13.848) (23.4886, 13.6734) (23.6632, 13.1695) (23.6632, 12.804) knots 0 0 0 1 2 2 2
  line L29 (23.6632, 12.804) -> (23.6632, 12.524)
  line L30 (23.6632, 12.524) -> (21.5521, 12.524)
  spline S51 degree 2 poles (21.5521, 12.524) (21.5521, 11.9938) (22.0856, 11.4306) (22.5599, 11.4306) knots 0 0 0 1 2 2 2
  spline S52 degree 2 poles (22.5599, 11.4306) (22.7279, 11.4306) (23.0539, 11.5064) (23.1856, 11.5657) knots 0 0 0 1 2 2 2
  spline S53 degree 2 poles (23.1856, 11.5657) (23.324, 11.6315) (23.515, 11.7468) (23.5775, 11.7995) knots 0 0 0 1 2 2 2
  line L31 (23.5775, 11.7995) -> (23.6072, 11.7995)
  line L32 (23.6072, 11.7995) -> (23.6072, 11.2396)
  spline S54 degree 2 poles (23.6072, 11.2396) (23.5183, 11.2034) (23.2482, 11.098) (23.1428, 11.0684) knots 0 0 0 1 2 2 2
  spline S55 degree 2 poles (23.1428, 11.0684) (22.9946, 11.0256) (22.7509, 10.9827) (22.5665, 10.9827) knots 0 0 0 1 2 2 2
  spline S56 degree 2 poles (23.1626, 12.9159) (23.156, 13.1234) (23.0704, 13.4264) (22.988, 13.5285) knots 0 0 0 1 2 2 2
  spline S57 degree 2 poles (22.988, 13.5285) (22.8991, 13.6438) (22.6192, 13.7656) (22.4117, 13.7656) knots 0 0 0 1 2 2 2
  spline S58 degree 2 poles (22.4117, 13.7656) (22.2075, 13.7656) (21.921, 13.6438) (21.8024, 13.5252) knots 0 0 0 1 2 2 2
  spline S59 degree 2 poles (21.8024, 13.5252) (21.6872, 13.4034) (21.5686, 13.1102) (21.5521, 12.9159) knots 0 0 0 1 2 2 2
  line L33 (21.5521, 12.9159) -> (23.1626, 12.9159)
  line L34 (26.5778, 11.0519) -> (26.064, 11.0519)
  line L35 (26.064, 11.0519) -> (26.064, 12.7908)
  spline S60 degree 2 poles (26.064, 12.7908) (26.064, 13.0016) (26.0245, 13.3638) (25.9652, 13.4725) knots 0 0 0 1 2 2 2
  spline S61 degree 2 poles (25.9652, 13.4725) (25.9026, 13.5878) (25.6787, 13.6998) (25.4877, 13.6998) knots 0 0 0 1 2 2 2
  spline S62 degree 2 poles (25.4877, 13.6998) (25.2967, 13.6998) (24.8916, 13.4956) (24.6973, 13.3309) knots 0 0 0 1 2 2 2
  line L36 (24.6973, 13.3309) -> (24.6973, 11.0519)
  line L37 (24.6973, 11.0519) -> (24.1835, 11.0519)
  line L38 (24.1835, 11.0519) -> (24.1835, 14.1015)
  line L39 (24.1835, 14.1015) -> (24.6973, 14.1015)
  line L40 (24.6973, 14.1015) -> (24.6973, 13.7623)
  spline S63 degree 2 poles (24.6973, 13.7623) (24.9278, 13.9698) (25.3724, 14.1872) (25.6227, 14.1872) knots 0 0 0 1 2 2 2
  spline S64 degree 2 poles (25.6227, 14.1872) (26.0706, 14.1872) (26.5778, 13.5944) (26.5778, 13.0312) knots 0 0 0 1 2 2 2
  line L41 (26.5778, 13.0312) -> (26.5778, 11.0519)
  spline S65 degree 2 poles (28.2212, 10.9926) (27.8029, 10.9926) (27.332, 11.4702) (27.332, 11.9872) knots 0 0 0 1 2 2 2
  line L42 (27.332, 11.9872) -> (27.332, 13.6767)
  line L43 (27.332, 13.6767) -> (26.9862, 13.6767)
  line L44 (26.9862, 13.6767) -> (26.9862, 14.1015)
  line L45 (26.9862, 14.1015) -> (27.332, 14.1015)
  line L46 (27.332, 14.1015) -> (27.332, 14.9776)
  line L47 (27.332, 14.9776) -> (27.8457, 14.9776)
  line L48 (27.8457, 14.9776) -> (27.8457, 14.1015)
  line L49 (27.8457, 14.1015) -> (28.7909, 14.1015)
  line L50 (28.7909, 14.1015) -> (28.7909, 13.6767)
  line L51 (28.7909, 13.6767) -> (27.8457, 13.6767)
  line L52 (27.8457, 13.6767) -> (27.8457, 12.2243)
  spline S66 degree 2 poles (27.8457, 12.2243) (27.8457, 11.9938) (27.8622, 11.7402) (27.9182, 11.6315) knots 0 0 0 1 2 2 2
  spline S67 degree 2 poles (27.9182, 11.6315) (27.9643, 11.536) (28.1718, 11.4405) (28.3496, 11.4405) knots 0 0 0 1 2 2 2
  spline S68 degree 2 poles (28.3496, 11.4405) (28.4748, 11.4405) (28.7086, 11.5163) (28.7613, 11.5393) knots 0 0 0 1 2 2 2
  line L53 (28.7613, 11.5393) -> (28.7909, 11.5393)
  line L54 (28.7909, 11.5393) -> (28.7909, 11.0782)
  spline S69 degree 2 poles (28.7909, 11.0782) (28.646, 11.0387) (28.3496, 10.9926) (28.2212, 10.9926) knots 0 0 0 1 2 2 2
  spline S70 degree 2 poles (33.3687, 13.0839) (33.3687, 11.9905) (32.7331, 10.9663) (32.0711, 10.9663) knots 0 0 0 1 2 2 2
  spline S71 degree 2 poles (32.0711, 10.9663) (31.3993, 10.9663) (30.7702, 12.0103) (30.7702, 13.0806) knots 0 0 0 1 2 2 2
  spline S72 degree 2 poles (30.7702, 13.0806) (30.7702, 14.1806) (31.4058, 15.1982) (32.0711, 15.1982) knots 0 0 0 1 2 2 2
  spline S73 degree 2 poles (32.0711, 15.1982) (32.7397, 15.1982) (33.3687, 14.1444) (33.3687, 13.0839) knots 0 0 0 1 2 2 2
  spline S74 degree 2 poles (32.6705, 11.8456) (32.7495, 12.0465) (32.8154, 12.6656) (32.8154, 13.0839) knots 0 0 0 1 2 2 2
  spline S75 degree 2 poles (32.8154, 13.0839) (32.8154, 13.5022) (32.7495, 14.118) (32.6672, 14.3255) knots 0 0 0 1 2 2 2
  spline S76 degree 2 poles (32.6672, 14.3255) (32.5849, 14.533) (32.2983, 14.747) (32.0711, 14.747) knots 0 0 0 1 2 2 2
  spline S77 degree 2 poles (32.0711, 14.747) (31.8439, 14.747) (31.5508, 14.533) (31.4651, 14.3189) knots 0 0 0 1 2 2 2
  spline S78 degree 2 poles (31.4651, 14.3189) (31.3828, 14.1114) (31.3235, 13.4791) (31.3235, 13.0806) knots 0 0 0 1 2 2 2
  spline S79 degree 2 poles (31.3235, 13.0806) (31.3235, 12.6525) (31.3762, 12.0794) (31.4618, 11.8555) knots 0 0 0 1 2 2 2
  spline S80 degree 2 poles (31.4618, 11.8555) (31.5409, 11.6447) (31.834, 11.4175) (32.0711, 11.4175) knots 0 0 0 1 2 2 2
  spline S81 degree 2 poles (32.0711, 11.4175) (32.295, 11.4175) (32.5882, 11.6315) (32.6705, 11.8456) knots 0 0 0 1 2 2 2
  line L55 (36.3953, 11.0519) -> (33.889, 11.0519)
  line L56 (33.889, 11.0519) -> (33.889, 11.6282)
  spline S82 degree 2 poles (33.889, 11.6282) (34.1591, 11.8818) (34.6399, 12.3528) (34.8705, 12.6064) knots 0 0 0 1 2 2 2
  spline S83 degree 2 poles (34.8705, 12.6064) (35.3348, 13.1168) (35.674, 13.7294) (35.674, 14.0554) knots 0 0 0 1 2 2 2
  spline S84 degree 2 poles (35.674, 14.0554) (35.674, 14.2267) (35.5686, 14.4836) (35.4731, 14.5659) knots 0 0 0 1 2 2 2
  spline S85 degree 2 poles (35.4731, 14.5659) (35.3776, 14.6482) (35.1273, 14.7306) (34.9758, 14.7306) knots 0 0 0 1 2 2 2
  spline S86 degree 2 poles (34.9758, 14.7306) (34.8309, 14.7306) (34.5345, 14.6581) (34.3995, 14.6021) knots 0 0 0 1 2 2 2
  spline S87 degree 2 poles (34.3995, 14.6021) (34.2842, 14.556) (34.0702, 14.4243) (34.0043, 14.3782) knots 0 0 0 1 2 2 2
  line L57 (34.0043, 14.3782) -> (33.9747, 14.3782)
  line L58 (33.9747, 14.3782) -> (33.9747, 14.9578)
  spline S88 degree 2 poles (33.9747, 14.9578) (34.1426, 15.0402) (34.7453, 15.2015) (35.0154, 15.2015) knots 0 0 0 1 2 2 2
  spline S89 degree 2 poles (35.0154, 15.2015) (35.5851, 15.2015) (36.2273, 14.5988) (36.2273, 14.0851) knots 0 0 0 1 2 2 2
  spline S90 degree 2 poles (36.2273, 14.0851) (36.2273, 13.8447) (36.1153, 13.4429) (36.0165, 13.2716) knots 0 0 0 1 2 2 2
  spline S91 degree 2 poles (36.0165, 13.2716) (35.9177, 13.0938) (35.6312, 12.7447) (35.4731, 12.5767) knots 0 0 0 1 2 2 2
  spline S92 degree 2 poles (35.4731, 12.5767) (35.2163, 12.2968) (34.5872, 11.6974) (34.3995, 11.5228) knots 0 0 0 1 2 2 2
  line L59 (34.3995, 11.5228) -> (36.3953, 11.5228)
  line L60 (36.3953, 11.5228) -> (36.3953, 11.0519)
  spline S93 degree 2 poles (12.2846, 7.1796) (12.2846, 6.9162) (12.0969, 6.4419) (11.9289, 6.2773) knots 0 0 0 1 2 2 2
  spline S94 degree 2 poles (11.9289, 6.2773) (11.7182, 6.0698) (11.1484, 5.8557) (10.7137, 5.8557) knots 0 0 0 1 2 2 2
  line L61 (10.7137, 5.8557) -> (10.2559, 5.8557)
  line L62 (10.2559, 5.8557) -> (10.2559, 4.3408)
  line L63 (10.2559, 4.3408) -> (9.7158, 4.3408)
  line L64 (9.7158, 4.3408) -> (9.7158, 8.4048)
  line L65 (9.7158, 8.4048) -> (10.7367, 8.4048)
  spline S95 degree 2 poles (10.7367, 8.4048) (11.099, 8.4048) (11.6062, 8.2862) (11.8005, 8.1512) knots 0 0 0 1 2 2 2
  spline S96 degree 2 poles (11.8005, 8.1512) (12.0277, 7.9964) (12.2846, 7.5189) (12.2846, 7.1796) knots 0 0 0 1 2 2 2
  spline S97 degree 2 poles (11.7215, 7.1632) (11.7215, 7.374) (11.5766, 7.6835) (11.4284, 7.7823) knots 0 0 0 1 2 2 2
  spline S98 degree 2 poles (11.4284, 7.7823) (11.2999, 7.868) (10.9574, 7.9371) (10.7038, 7.9371) knots 0 0 0 1 2 2 2
  line L66 (10.7038, 7.9371) -> (10.2559, 7.9371)
  line L67 (10.2559, 7.9371) -> (10.2559, 6.3168)
  line L68 (10.2559, 6.3168) -> (10.6248, 6.3168)
  spline S99 degree 2 poles (10.6248, 6.3168) (10.9541, 6.3168) (11.3592, 6.4222) (11.4909, 6.5605) knots 0 0 0 1 2 2 2
  spline S100 degree 2 poles (11.4909, 6.5605) (11.6128, 6.6824) (11.7215, 6.9689) (11.7215, 7.1632) knots 0 0 0 1 2 2 2
  line L69 (14.3759, 6.8404) -> (14.3496, 6.8404)
  spline S101 degree 2 poles (14.3496, 6.8404) (14.2903, 6.8569) (14.1618, 6.8635) (14.0729, 6.8635) knots 0 0 0 1 2 2 2
  spline S102 degree 2 poles (14.0729, 6.8635) (13.8654, 6.8635) (13.4571, 6.6824) (13.2726, 6.5045) knots 0 0 0 1 2 2 2
  line L70 (13.2726, 6.5045) -> (13.2726, 4.3408)
  line L71 (13.2726, 4.3408) -> (12.7589, 4.3408)
  line L72 (12.7589, 4.3408) -> (12.7589, 7.3904)
  line L73 (12.7589, 7.3904) -> (13.2726, 7.3904)
  line L74 (13.2726, 7.3904) -> (13.2726, 6.9359)
  spline S103 degree 2 poles (13.2726, 6.9359) (13.5526, 7.1862) (13.9708, 7.3904) (14.1684, 7.3904) knots 0 0 0 1 2 2 2
  spline S104 degree 2 poles (14.1684, 7.3904) (14.2475, 7.3904) (14.3265, 7.3838) (14.3759, 7.374) knots 0 0 0 1 2 2 2
  line L75 (14.3759, 7.374) -> (14.3759, 6.8404)
  line L76 (15.298, 4.3408) -> (14.7843, 4.3408)
  line L77 (14.7843, 4.3408) -> (14.7843, 7.3904)
  line L78 (14.7843, 7.3904) -> (15.298, 7.3904)
  line L79 (15.298, 7.3904) -> (15.298, 4.3408)
  line L80 (15.3343, 7.8976) -> (14.7513, 7.8976)
  line L81 (14.7513, 7.8976) -> (14.7513, 8.4311)
  line L82 (14.7513, 8.4311) -> (15.3343, 8.4311)
  line L83 (15.3343, 8.4311) -> (15.3343, 7.8976)
  line L84 (18.4465, 4.3408) -> (17.9327, 4.3408)
  line L85 (17.9327, 4.3408) -> (17.9327, 6.0797)
  spline S105 degree 2 poles (17.9327, 6.0797) (17.9327, 6.2904) (17.8932, 6.6527) (17.8339, 6.7614) knots 0 0 0 1 2 2 2
  spline S106 degree 2 poles (17.8339, 6.7614) (17.7714, 6.8767) (17.5474, 6.9886) (17.3564, 6.9886) knots 0 0 0 1 2 2 2
  spline S107 degree 2 poles (17.3564, 6.9886) (17.1654, 6.9886) (16.7603, 6.7844) (16.566, 6.6198) knots 0 0 0 1 2 2 2
  line L86 (16.566, 6.6198) -> (16.566, 4.3408)
  line L87 (16.566, 4.3408) -> (16.0522, 4.3408)
  line L88 (16.0522, 4.3408) -> (16.0522, 7.3904)
  line L89 (16.0522, 7.3904) -> (16.566, 7.3904)
  line L90 (16.566, 7.3904) -> (16.566, 7.0512)
  spline S108 degree 2 poles (16.566, 7.0512) (16.7965, 7.2587) (17.2411, 7.476) (17.4914, 7.476) knots 0 0 0 1 2 2 2
  spline S109 degree 2 poles (17.4914, 7.476) (17.9393, 7.476) (18.4465, 6.8832) (18.4465, 6.3201) knots 0 0 0 1 2 2 2
  line L91 (18.4465, 6.3201) -> (18.4465, 4.3408)
  spline S110 degree 2 poles (20.0899, 4.2815) (19.6716, 4.2815) (19.2007, 4.759) (19.2007, 5.2761) knots 0 0 0 1 2 2 2
  line L92 (19.2007, 5.2761) -> (19.2007, 6.9656)
  line L93 (19.2007, 6.9656) -> (18.8549, 6.9656)
  line L94 (18.8549, 6.9656) -> (18.8549, 7.3904)
  line L95 (18.8549, 7.3904) -> (19.2007, 7.3904)
  line L96 (19.2007, 7.3904) -> (19.2007, 8.2665)
  line L97 (19.2007, 8.2665) -> (19.7144, 8.2665)
  line L98 (19.7144, 8.2665) -> (19.7144, 7.3904)
  line L99 (19.7144, 7.3904) -> (20.6596, 7.3904)
  line L100 (20.6596, 7.3904) -> (20.6596, 6.9656)
  line L101 (20.6596, 6.9656) -> (19.7144, 6.9656)
  line L102 (19.7144, 6.9656) -> (19.7144, 5.5132)
  spline S111 degree 2 poles (19.7144, 5.5132) (19.7144, 5.2827) (19.7309, 5.0291) (19.7869, 4.9204) knots 0 0 0 1 2 2 2
  spline S112 degree 2 poles (19.7869, 4.9204) (19.833, 4.8249) (20.0405, 4.7294) (20.2183, 4.7294) knots 0 0 0 1 2 2 2
  spline S113 degree 2 poles (20.2183, 4.7294) (20.3435, 4.7294) (20.5773, 4.8051) (20.63, 4.8282) knots 0 0 0 1 2 2 2
  line L103 (20.63, 4.8282) -> (20.6596, 4.8282)
  line L104 (20.6596, 4.8282) -> (20.6596, 4.3671)
  spline S114 degree 2 poles (20.6596, 4.3671) (20.5147, 4.3276) (20.2183, 4.2815) (20.0899, 4.2815) knots 0 0 0 1 2 2 2
  line L105 (25.7709, 8.4048) -> (24.3712, 4.3408)
  line L106 (24.3712, 4.3408) -> (23.7883, 4.3408)
  line L107 (23.7883, 4.3408) -> (22.3886, 8.4048)
  line L108 (22.3886, 8.4048) -> (22.9683, 8.4048)
  line L109 (22.9683, 8.4048) -> (24.0946, 5.0291)
  line L110 (24.0946, 5.0291) -> (25.2209, 8.4048)
  line L111 (25.2209, 8.4048) -> (25.7709, 8.4048)
  line L112 (27.579, 5.8722) -> (26.041, 5.8722)
  line L113 (26.041, 5.8722) -> (26.041, 6.3662)
  line L114 (26.041, 6.3662) -> (27.579, 6.3662)
  line L115 (27.579, 6.3662) -> (27.579, 5.8722)
  spline S115 degree 2 poles (30.6484, 6.3728) (30.6484, 5.2794) (30.0128, 4.2551) (29.3508, 4.2551) knots 0 0 0 1 2 2 2
  spline S116 degree 2 poles (29.3508, 4.2551) (28.6789, 4.2551) (28.0499, 5.2991) (28.0499, 6.3695) knots 0 0 0 1 2 2 2
  spline S117 degree 2 poles (28.0499, 6.3695) (28.0499, 7.4695) (28.6855, 8.4871) (29.3508, 8.4871) knots 0 0 0 1 2 2 2
  spline S118 degree 2 poles (29.3508, 8.4871) (30.0193, 8.4871) (30.6484, 7.4332) (30.6484, 6.3728) knots 0 0 0 1 2 2 2
  spline S119 degree 2 poles (29.9502, 5.1345) (30.0292, 5.3354) (30.0951, 5.9545) (30.0951, 6.3728) knots 0 0 0 1 2 2 2
  spline S120 degree 2 poles (30.0951, 6.3728) (30.0951, 6.791) (30.0292, 7.4069) (29.9469, 7.6144) knots 0 0 0 1 2 2 2
  spline S121 degree 2 poles (29.9469, 7.6144) (29.8646, 7.8219) (29.578, 8.0359) (29.3508, 8.0359) knots 0 0 0 1 2 2 2
  spline S122 degree 2 poles (29.3508, 8.0359) (29.1235, 8.0359) (28.8304, 7.8219) (28.7448, 7.6078) knots 0 0 0 1 2 2 2
  spline S123 degree 2 poles (28.7448, 7.6078) (28.6625, 7.4003) (28.6032, 6.768) (28.6032, 6.3695) knots 0 0 0 1 2 2 2
  spline S124 degree 2 poles (28.6032, 6.3695) (28.6032, 5.9413) (28.6559, 5.3683) (28.7415, 5.1444) knots 0 0 0 1 2 2 2
  spline S125 degree 2 poles (28.7415, 5.1444) (28.8206, 4.9336) (29.1137, 4.7063) (29.3508, 4.7063) knots 0 0 0 1 2 2 2
  spline S126 degree 2 poles (29.3508, 4.7063) (29.5747, 4.7063) (29.8678, 4.9204) (29.9502, 5.1345) knots 0 0 0 1 2 2 2
  line L116 (33.675, 4.3408) -> (31.1687, 4.3408)
  line L117 (31.1687, 4.3408) -> (31.1687, 4.9171)
  spline S127 degree 2 poles (31.1687, 4.9171) (31.4388, 5.1707) (31.9196, 5.6417) (32.1501, 5.8952) knots 0 0 0 1 2 2 2
  spline S128 degree 2 poles (32.1501, 5.8952) (32.6145, 6.4057) (32.9537, 7.0183) (32.9537, 7.3443) knots 0 0 0 1 2 2 2
  spline S129 degree 2 poles (32.9537, 7.3443) (32.9537, 7.5156) (32.8483, 7.7725) (32.7528, 7.8548) knots 0 0 0 1 2 2 2
  spline S130 degree 2 poles (32.7528, 7.8548) (32.6573, 7.9371) (32.407, 8.0195) (32.2555, 8.0195) knots 0 0 0 1 2 2 2
  spline S131 degree 2 poles (32.2555, 8.0195) (32.1106, 8.0195) (31.8142, 7.947) (31.6792, 7.891) knots 0 0 0 1 2 2 2
  spline S132 degree 2 poles (31.6792, 7.891) (31.5639, 7.8449) (31.3499, 7.7132) (31.284, 7.6671) knots 0 0 0 1 2 2 2
  line L118 (31.284, 7.6671) -> (31.2544, 7.6671)
  line L119 (31.2544, 7.6671) -> (31.2544, 8.2467)
  spline S133 degree 2 poles (31.2544, 8.2467) (31.4223, 8.329) (32.025, 8.4904) (32.2951, 8.4904) knots 0 0 0 1 2 2 2
  spline S134 degree 2 poles (32.2951, 8.4904) (32.8648, 8.4904) (33.507, 7.8877) (33.507, 7.374) knots 0 0 0 1 2 2 2
  spline S135 degree 2 poles (33.507, 7.374) (33.507, 7.1335) (33.395, 6.7318) (33.2962, 6.5605) knots 0 0 0 1 2 2 2
  spline S136 degree 2 poles (33.2962, 6.5605) (33.1974, 6.3827) (32.9109, 6.0336) (32.7528, 5.8656) knots 0 0 0 1 2 2 2
  spline S137 degree 2 poles (32.7528, 5.8656) (32.4959, 5.5857) (31.8669, 4.9863) (31.6792, 4.8117) knots 0 0 0 1 2 2 2
  line L120 (31.6792, 4.8117) -> (33.675, 4.8117)
  line L121 (33.675, 4.8117) -> (33.675, 4.3408)
  constraints: 4 end point, 2 midpoint, 1 horizontal, 1 perpendicular, 1 point on line
extrude "Extrusion12" cut sketch "Sketch12" against normal blind 1.27
equation "\"partDepth\" = 20.32"
equation "\"partWidth\" = 86.36"
body "Solid2"
